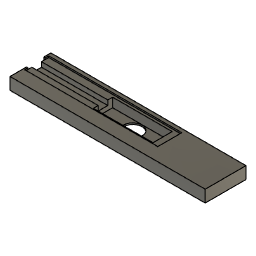
Easel base (CNC wood) (Autodesk Fusion 360 design; units mm, degrees)
Autodesk Fusion 360 part; units mm, degrees
sketch "Sketch1" plane through (0, 0, 0) normal (0, 0, 1) x (1, 0, 0)
  line L0 (0, 0) -> (125, 0) construction
  line L1 (125, 0) -> (125, 40) construction
  line L2 (125, 40) -> (0, 40) construction
  line L3 (0, 40) -> (0, 0) construction
  line L4 (-140.7, 62.5) -> (265.7, 62.5)
  line L5 (265.7, 62.5) -> (265.7, -22.5)
  line L6 (265.7, -22.5) -> (-140.7, -22.5)
  line L7 (-140.7, -22.5) -> (-140.7, 62.5)
  line L8 (-140.7, 20) -> (265.7, 20) construction
  line L9 (62.5, 62.5) -> (62.5, -22.5) construction
  point P0 (125, 20)
  point P1 (62.5, 40)
  dimension "d1" = 125
  dimension "d2" = 40
  dimension "d3" = 85
  dimension "d4" = 406.4
  constraint horizontal L0
  constraint vertical L1
  constraint horizontal L2
  constraint vertical L3
  constraint coincident L0.start L3.end
  constraint horizontal L4
  constraint vertical L5
  constraint horizontal L6
  constraint vertical L7
  constraint midpoint L7 L8.start
  constraint midpoint L5 L8.end
  constraint midpoint L1 P0
  constraint coincident L8 P0
  constraint midpoint L4 L9.start
  constraint midpoint L6 L9.end
  constraint midpoint L2 P1
  constraint coincident L9 P1
  measures "d1" distance of L0.start L0.end
  measures "d2" distance of L0.start L2.end
  measures "d3" distance of L9.start L9.end
  measures "d4" distance of L5.end L6.end L0.start
extrude "Extrude1" add sketch "Sketch1" along normal blind 25 makes body 1
sketch "Sketch2" plane through (0, 0, 25) normal (0, 0, 1) x (-1, 0, 0)
  line L0 (140.7, 22.5) -> (-265.7, 22.5)
  line L1 (-265.7, 22.5) -> (-265.7, -62.5)
  line L2 (-265.7, -62.5) -> (140.7, -62.5)
  line L3 (140.7, -62.5) -> (140.7, 22.5)
  line L4 (140.7, -62.5) -> (-265.7, 22.5) construction
  line L5 (-265.7, -62.5) -> (140.7, 22.5) construction
  line L6 (-124.5, 0) -> (-0.5, 0)
  line L7 (-0.5, 0) -> (-0.5, -40)
  line L8 (-0.5, -40) -> (-124.5, -40)
  line L9 (-124.5, -40) -> (-124.5, 0)
  line L10 (-124.5, 0) -> (-0.5, -40) construction
  line L11 (-0.5, 0) -> (-124.5, -40) construction
  point P0 (-62.5, -20)
  dimension "d7" = 124
  dimension "d8" = 40
  constraint coincident L2.end L3.start
  constraint coincident L0.end L1.start
  constraint coincident L1.end L2.start
  constraint coincident L0.start L3.end
  constraint perpendicular L6 L7
  constraint parallel L6 L8
  constraint parallel L7 L9
  constraint horizontal L6
  constraint coincident L10 P0
  constraint coincident L11 P0
  constraint midpoint L4 P0
  measures "d7" distance of L7.end L8.end
  measures "d8" distance of L6.start L8.end
extrude "Extrude2" cut sketch "Sketch2" against normal up to surface (22 mm away) contours L6 L7 L8 L9 bodies 1
sketch "Sketch3" plane through (0, 0, 3) normal (0, 0, 1) x (-1, 0, 0)
  line L0 (-0.5, -40) -> (-0.5, 0)
  line L1 (-0.5, 0) -> (-124.5, 0)
  line L2 (-124.5, 0) -> (-124.5, -40)
  line L3 (-124.5, -40) -> (-0.5, -40)
  line L4 (-62.5, -40) -> (-62.5, 0) construction
  circle A0 centre (-62.5, -20) radius 19.5
  point P0 (-62.5, -40)
  point P1 (-62.5, 0)
  dimension "d31" = 39
  constraint midpoint L3 P0
  constraint midpoint L1 P1
  constraint coincident P0 L4.start
  constraint coincident P1 L4.end
  constraint midpoint L4 A0.centre
  measures "d31" diameter of A0
extrude "Extrude3" cut sketch "Sketch3" against normal up to surface (3 mm away) contours A0 bodies 1
sketch "Sketch6" plane through (-140.7, 0, 0) normal (-1, 0, 0) x (0, -1, 0)
  line L0 (-62.5, 0) -> (22.5, 0)
  line L1 (22.5, 0) -> (22.5, 25)
  line L2 (22.5, 25) -> (-62.5, 25)
  line L3 (-62.5, 25) -> (-62.5, 0)
  line L4 (-30, 25) -> (-10, 25)
  line L5 (-10, 25) -> (-10, 12)
  line L6 (-10, 12) -> (-30, 12)
  line L7 (-30, 12) -> (-30, 25)
  point P0 (-20, 25)
  dimension "d17" = 13
  dimension "d18" = 20
  constraint horizontal L4
  constraint vertical L5
  constraint horizontal L6
  constraint vertical L7
  constraint coincident L2 L4.start
  constraint midpoint L4 P0
  constraint midpoint L2 P0
  measures "d17" distance of L4.start L6.end
  measures "d18" distance of L4.start L4.end
extrude "Extrude5" cut sketch "Sketch6" against normal up to surface (265.2 mm away) contours L2 L4 L5 L6 L7 bodies 1
sketch "Sketch7" plane through (-140.7, 0, 0) normal (-1, 0, 0) x (0, -1, 0)
  line L0 (-30, 12) -> (-30, 25)
  line L1 (-30, 25) -> (-62.5, 25)
  line L2 (-62.5, 25) -> (-62.5, 0)
  line L3 (-62.5, 0) -> (22.5, 0)
  line L4 (22.5, 0) -> (22.5, 25)
  line L5 (22.5, 25) -> (-10, 25)
  line L6 (-10, 25) -> (-10, 12)
  line L7 (-10, 12) -> (-30, 12)
  line L8 (-38, 25) -> (-2, 25)
  line L9 (-2, 25) -> (-2, 9)
  line L10 (-2, 9) -> (-38, 9)
  line L11 (-38, 9) -> (-38, 25)
  line L12 (-20, 12) -> (-20, 9) construction
  dimension "d21" = 3
  dimension "d22" = 8
  constraint horizontal L8
  constraint vertical L9
  constraint horizontal L10
  constraint vertical L11
  constraint coincident L1 L8.start
  constraint midpoint L7 L12.start
  constraint midpoint L10 L12.end
  constraint vertical L12
  measures "d21" distance of L7 L10
  measures "d22" distance of L0 L11
extrude "Extrude6" cut sketch "Sketch7" against normal blind 3 contours L0 L1 L5 L6 L7 L8 L9 L10 L11 bodies 1
sketch "Sketch8" plane through (0, 0, 25) normal (0, 0, 1) x (-1, 0, 0)
  line L0 (140.7, -38) -> (137.7, -38)
  line L1 (137.7, -38) -> (137.7, -30)
  line L2 (137.7, -30) -> (-0.5, -30)
  line L3 (-0.5, -30) -> (-0.5, -40)
  line L4 (-0.5, -40) -> (-124.5, -40)
  line L5 (-124.5, -40) -> (-124.5, 0)
  line L6 (-124.5, 0) -> (-0.5, 0)
  line L7 (-0.5, 0) -> (-0.5, -10)
  line L8 (-0.5, -10) -> (137.7, -10)
  line L9 (137.7, -10) -> (137.7, -2)
  line L10 (137.7, -2) -> (140.7, -2)
  line L11 (140.7, -2) -> (140.7, 22.5)
  curve K0
  line L12 (-265.7, 22.5) -> (-265.7, -62.5)
  line L13 (-265.7, -62.5) -> (140.7, -62.5)
  line L14 (140.7, -62.5) -> (140.7, -38)
  line L15 (-139.5, -45) -> (137.7, -45)
  line L16 (137.7, -45) -> (137.7, 5)
  line L17 (137.7, 5) -> (-139.5, 5)
  line L18 (-139.5, 5) -> (-139.5, -45)
  line L19 (-124.5, -20) -> (-139.5, -20) construction
  dimension "d25" = 5
  dimension "d26" = 15
  constraint horizontal L15
  constraint vertical L16
  constraint horizontal L17
  constraint vertical L18
  constraint coincident L1.end L16
  constraint midpoint L5 L19.start
  constraint midpoint L18 L19.end
  constraint horizontal L19
  measures "d25" distance of L6 L17
  measures "d26" distance of L5 L18
extrude "Extrude7" cut sketch "Sketch8" against normal blind 3 contours L1 L2 L3 L4 L5 L6 L7 L8 L9 L15 L16 L17 L18 bodies 1
extrude "Extrude8" add 1 faces at (-79.4667, 20, 0) along direction (0, 0, 1) blind 38.1 separate body on bodies 1 makes body 2
move_face "OffsetFaces1" offset -10 1 faces at (-5.2333, 62.5, 8.3333) on bodies 1
move_face "OffsetFaces2" offset 10 1 faces at (130.2333, -22.5, 8.3333) on bodies 1
hidden bodies 2
